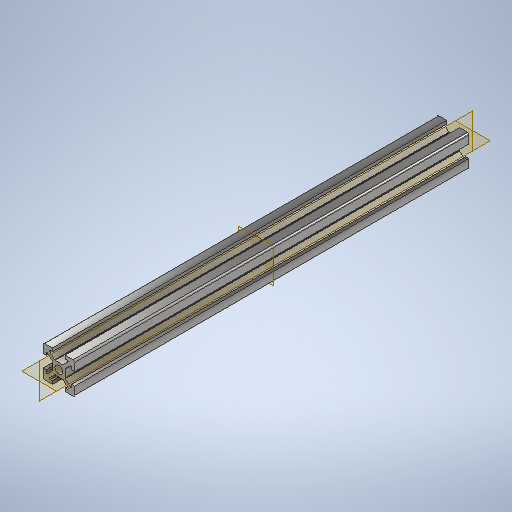
# Autodesk Inventor part: Ext_001
Saved by Autodesk Inventor 2025.2 (Build 292293000, 293)
## iProperties
Created: 2025-03-25
Part Number: Ext_001
Material: Aço galvanizado
Document SubType Name: Modeling
Designer: Formação
Density: 7.85 g/cm^3
Appearance: Semipolido
Author: Formação
Autodesk Inventor part; units mm, degrees
sketch "Esboço1" plane through (0, 0, 0) normal (0, 0, 1) x (1, 0, 0)
  line L0 (-10, 10) -> (10, 10) construction
  circle A0 centre (0, 0) radius 2.5 construction
  line L1 (-4, 4) -> (4, 4) construction
  line L2 (-4, 4) -> (-4, -4) construction
  line L3 (-10, 10) -> (0, 0) construction
  line L4 (-2.5858, 4) -> (-6.5858, 8) construction
  line L5 (-6.5858, 8) -> (0, 8) construction
  arc A1 (-5.3787, 8) -> (-5.7322, 7.1464) centre (-5.3787, 7.5) ccw
  arc A2 (-2.7322, 4.1464) -> (-2.3787, 4) centre (-2.3787, 4.5) ccw
  line L6 (0, 4) -> (-4, 4) construction
  line L7 (-2.3787, 4) -> (0, 4)
  line L8 (-4, 10) -> (-4, 8) construction
  line L9 (-5.3787, 8) -> (-4, 8)
  line L10 (-5.7322, 7.1464) -> (-2.7322, 4.1464)
  line L11 (-4, 10) -> (-4, 9) construction
  line L12 (-4, 9) -> (-4, 9) construction
  line L13 (-4, 10) -> (-4, 9)
  line L14 (-4, 9) -> (-4, 9)
  line L15 (-4, 9) -> (-4, 8)
  line L16 (0, 4) -> (0, 2.5)
  arc A3 (-9, 10) -> (-9.7071, 9.7071) centre (-9, 9) ccw
  line L17 (-9, 10) -> (-4, 10)
  line L18 (-9.7071, 9.7071) -> (-1.7678, 1.7678)
  arc A4 (0, 2.5) -> (-1.7678, 1.7678) centre (0, 0) ccw
  line L19 (-4, 10) -> (-9, 10)
  line L20 (10, 10) -> (10, -10) construction
  line L21 (10, 10) -> (30, 10) construction
  line L22 (20, 10) -> (20, -10) construction
  arc A5 (25.7322, 7.1464) -> (25.3787, 8) centre (25.3787, 7.5) ccw
  arc A6 (22.3787, 4) -> (22.7322, 4.1464) centre (22.3787, 4.5) ccw
  line L23 (22.3787, 4) -> (20, 4)
  line L24 (25.3787, 8) -> (24, 8)
  line L25 (25.7322, 7.1464) -> (22.7322, 4.1464)
  line L26 (24, 10) -> (24, 9)
  line L27 (24, 9) -> (24, 8)
  line L28 (20, 4) -> (20, 2.5)
  arc A7 (29.7071, 9.7071) -> (29, 10) centre (29, 9) ccw
  line L29 (29.7071, 9.7071) -> (21.7678, 1.7678)
  line L30 (24, 10) -> (29, 10)
  line L31 (10, 0) -> (30, 0) construction
  line L32 (29.7071, -9.7071) -> (21.7678, -1.7678)
  line L33 (25.7322, -7.1464) -> (22.7322, -4.1464)
  line L34 (24, -10) -> (29, -10)
  line L35 (24, -10) -> (24, -9)
  line L36 (24, -9) -> (24, -8)
  line L37 (25.3787, -8) -> (24, -8)
  arc A8 (17.2678, 4.1464) -> (17.6213, 4) centre (17.6213, 4.5) ccw
  line L38 (17.6213, 4) -> (20, 4)
  arc A9 (29, -10) -> (29.7071, -9.7071) centre (29, -9) ccw
  arc A10 (25.3787, -8) -> (25.7322, -7.1464) centre (25.3787, -7.5) ccw
  arc A11 (22.7322, -4.1464) -> (22.3787, -4) centre (22.3787, -4.5) ccw
  line L39 (22.3787, -4) -> (20, -4)
  line L40 (20, -4) -> (20, -2.5)
  arc A12 (29.7071, 9.7071) -> (29, 10) centre (29, 9) ccw
  line L41 (30, 0) -> (30, -10) construction
  line L42 (16, 10) -> (16, 9)
  line L43 (16, 9) -> (16, 8)
  line L44 (14.6213, 8) -> (16, 8)
  arc A13 (14.6213, 8) -> (14.2678, 7.1464) centre (14.6213, 7.5) ccw
  line L45 (14.2678, 7.1464) -> (17.2678, 4.1464)
  line L46 (10.2929, 9.7071) -> (18.2322, 1.7678)
  line L47 (16, 10) -> (11, 10)
  arc A14 (11, 10) -> (10.2929, 9.7071) centre (11, 9) ccw
  circle A15 centre (20, 0) radius 2.5
  arc A16 (29.7071, 9.7071) -> (29, 10) centre (29, 9) ccw
  arc A17 (29, -10) -> (29.7071, -9.7071) centre (29, -9) ccw
  line L48 (27.1464, -5.7322) -> (24.1464, -2.7322)
  line L49 (27.1464, -5.7322) -> (24.1464, -2.7322)
  line L50 (28, -5.3787) -> (28, -4)
  line L51 (30, -4) -> (29, -4)
  line L52 (29, -4) -> (28, -4)
  line L53 (30, -4) -> (30, -9)
  arc A18 (29.7071, -9.7071) -> (30, -9) centre (29, -9) ccw
  arc A19 (27.1464, -5.7322) -> (28, -5.3787) centre (27.5, -5.3787) ccw
  arc A20 (24, -2.3787) -> (24.1464, -2.7322) centre (24.5, -2.3787) ccw
  line L54 (24, -2.3787) -> (24, 0)
  line L55 (24, 0) -> (22.5, 0)
  line L56 (30, 4) -> (30, 9)
  arc A21 (30, 9) -> (29.7071, 9.7071) centre (29, 9) ccw
  line L57 (30, 4) -> (29, 4)
  line L58 (29, 4) -> (28, 4)
  line L59 (28, 5.3787) -> (28, 4)
  arc A22 (28, 5.3787) -> (27.1464, 5.7322) centre (27.5, 5.3787) ccw
  line L60 (27.1464, 5.7322) -> (24.1464, 2.7322)
  arc A23 (24.1464, 2.7322) -> (24, 2.3787) centre (24.5, 2.3787) ccw
  line L61 (24, 2.3787) -> (24, 0)
  line L62 (24, 0) -> (22.5, 0)
  line L63 (16, 0) -> (17.5, 0)
  line L64 (16, 2.3787) -> (16, 0)
  arc A24 (16, 2.3787) -> (15.8536, 2.7322) centre (15.5, 2.3787) ccw
  line L65 (12.8536, 5.7322) -> (15.8536, 2.7322)
  arc A25 (12.8536, 5.7322) -> (12, 5.3787) centre (12.5, 5.3787) ccw
  line L66 (12, 5.3787) -> (12, 4)
  line L67 (11, 4) -> (12, 4)
  line L68 (10, 4) -> (11, 4)
  line L69 (10, 4) -> (10, 9)
  arc A26 (10.2929, 9.7071) -> (10, 9) centre (11, 9) ccw
  line L70 (10.2929, -9.7071) -> (18.2322, -1.7678)
  line L71 (16, -2.3787) -> (16, 0)
  line L72 (12.8536, -5.7322) -> (15.8536, -2.7322)
  arc A27 (15.8536, -2.7322) -> (16, -2.3787) centre (15.5, -2.3787) ccw
  arc A28 (12, -5.3787) -> (12.8536, -5.7322) centre (12.5, -5.3787) ccw
  line L73 (12, -5.3787) -> (12, -4)
  line L74 (11, -4) -> (12, -4)
  line L75 (10, -4) -> (11, -4)
  line L76 (10, -4) -> (10, -9)
  arc A29 (10, -9) -> (10.2929, -9.7071) centre (11, -9) ccw
  line L77 (30, -10) -> (10, -10) construction
  line L78 (20, -4) -> (20, -2.5)
  line L79 (14.2678, -7.1464) -> (17.2678, -4.1464)
  arc A30 (17.6213, -4) -> (17.2678, -4.1464) centre (17.6213, -4.5) ccw
  line L80 (17.6213, -4) -> (20, -4)
  line L81 (14.6213, -8) -> (16, -8)
  arc A31 (14.2678, -7.1464) -> (14.6213, -8) centre (14.6213, -7.5) ccw
  line L82 (16, -9) -> (16, -8)
  line L83 (16, -10) -> (16, -9)
  line L84 (16, -10) -> (11, -10)
  arc A32 (10.2929, -9.7071) -> (11, -10) centre (11, -9) ccw
  line L85 (0, 10) -> (0, -11) construction
  line L86 (10, 0) -> (-11, 0) construction
  arc A33 (-4, 2.3787) -> (-4.1464, 2.7322) centre (-4.5, 2.3787) ccw
  line L87 (-4, 0) -> (-2.5, 0)
  arc A34 (-1.7678, 1.7678) -> (-2.5, 0) centre (0, 0) ccw
  point P0 (-5, 5)
  point P1 (-5.8406, 7.6913)
  point P2 (-9.3827, 9.9239)
  point P3 (-6.5, 10)
  point P4 (-4, 2.5858)
  dimension "d1" = 10
  dimension "d2" = 5
  dimension "d5" = 20
  dimension "d10" = 1
  dimension "d11" = 2
  dimension "d17" = 6
  dimension "d18" = 0.5
  dimension "d24" = 1
  dimension "d25" = 0.5
  dimension "d41" = 20
  dimension "d42" = 20
  dimension "d43" = 20
  dimension "d46" = 10
  dimension "d47" = 10
  constraints: 176 end point, 121 symmetric about line, 70 point on circle, 34 centre point, 10 midpoint, 9 horizontal, 9 point on line, 6 collinear, 6 vertical, 5 tangent, 5 vertical alignment, 4 perpendicular, 3 horizontal alignment, 2 coincident, 1 line through centre, 1 parallel, 32 other
  measures "d1" horizontal distance of point (0, 0) L0.start
  measures "d2" diameter of A0
  measures "d5" distance of L0.end L0.start
  measures "d10" distance from line of point (-5, 5) L4
  measures "d11" distance from line of L4.end L0
  measures "d17" distance between parallel lines of L0 L1
  measures "d18" radius of A2
  measures "d24" radius of A3
  measures "d25" radius of A1
  measures "d41" distance of L0.end L20.end
  measures "d42" distance of L0.end L21.end
  measures "d43" distance of L22.start L22.end
  measures "d46" distance of L22.end L41.end
  measures "d47" distance of L31.end L41.end
extrude "Extrusão1" add sketch "Esboço1" along normal mid plane 250 contours A1 L10 A2 L7 L16 A4 L18 A3 L17 L13 L15 L9
mirror "Espelhar1" about plane through (-9.7071, 9.7071, 0) normal (-0.7071, -0.7071, 0)
mirror "Espelhar2" about plane through (0, 0, 0) normal (1, 0, 0)
mirror "Espelhar3" about plane through (0, 0, 0) normal (0, 1, 0)
